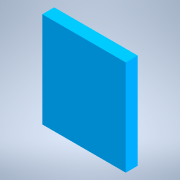
# Autodesk Inventor part: ToF Sensor7
Saved by Autodesk Inventor 2022.3 (Build 263350000, 350)
## iProperties
Created: 2023-02-07
Part Number: ToF Sensor7
Material: Generic
Document SubType Name: Modeling
Designer: lbmcgill42
Density: 1 g/cm^3
Appearance: Default
Author: lbmcgill42
Autodesk Inventor part; units mm, degrees
ref_plane "YZ Plane" through (0, 0, 0) normal (1, 0, 0) x (0, 1, 0)
ref_plane "XZ Plane" through (0, 0, 0) normal (0, 1, 0) x (-1, 0, 0)
ref_plane "XY Plane" through (0, 0, 0) normal (0, 0, 1) x (1, 0, 0)
sketch "Sketch1" plane through (0, 0, 0) normal (0, 0, 1) x (1, 0, 0)
  line L0 (-26.2497, 19.4793) -> (-8.4697, 19.4793)
  line L1 (-8.4697, 19.4793) -> (-8.4697, -0.8407)
  line L2 (-8.4697, -0.8407) -> (-26.2497, -0.8407)
  line L3 (-26.2497, -0.8407) -> (-26.2497, 19.4793)
  point P0 (0, 0)
  dimension "d0" = 17.78
  dimension "d1" = 20.32
  constraints: 8 end point, 2 parallel, 1 horizontal, 1 perpendicular
  measures "d0" distance of L1.end L2.end
  measures "d1" distance of L0.end L1.end
extrude "Extrusion1" add sketch "Sketch1" along normal blind 2.54
body "Solid1"
